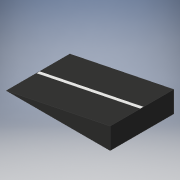
# Autodesk Inventor part: Ramp
Saved by Autodesk Inventor 2017 (Build 210142000, 142)
## iProperties
Created: 2017-04-14
Part Number: Ramp
Material: Generic
Document SubType Name: Modeling
Designer: Alex Tacescu
Density: 1 g/cm^3
Appearance: Rubber - Black
Author: Alex Tacescu
Autodesk Inventor part; units mm, degrees
ref_plane "YZ Plane" through (0, 0, 0) normal (1, 0, 0) x (0, 1, 0)
ref_plane "XZ Plane" through (0, 0, 0) normal (0, 1, 0) x (-1, 0, 0)
ref_plane "XY Plane" through (0, 0, 0) normal (0, 0, 1) x (1, 0, 0)
sketch "Sketch1" plane through (0, 0, 0) normal (0, 0, 1) x (1, 0, 0)
  line L0 (0, 0) -> (746.6045, 152.4)
  line L1 (0, 182.88) -> (0, -30.48) projected
  line L2 (-149.3209, 0) -> (895.9254, 0) projected
  line L3 (746.6045, 152.4) -> (746.6045, 0)
  line L4 (0, 0) -> (746.6045, 0)
  dimension "d0" = 152.4
  dimension "d1" = 762
  constraints: 6 end point, 1 perpendicular, 1 point on line, 1 vertical
  measures "d0" distance of L0.end L3.end
  measures "d1" distance of L0.start L0.end
extrude "Extrusion1" add sketch "Sketch1" along normal mid plane 457.2
sketch "Sketch4" plane through (0, 0, 228.6) normal (-0.2, 0.9798, 0) x (0.9798, 0.2, 0)
  line L0 (914.4, 228.6) -> (-152.4, 228.6) projected
  line L1 (762, 215.9) -> (0, 215.9)
  line L2 (0, 215.9) -> (0, 241.3)
  line L3 (0, 241.3) -> (762, 241.3)
  line L4 (762, 241.3) -> (762, 215.9)
  line L5 (762, 215.9) -> (0, 241.3) construction
  line L6 (0, 215.9) -> (762, 241.3) construction
  line L7 (0, 0) -> (0, 457.2) projected
  line L8 (762, 0) -> (0, 0) projected
  line L9 (762, 457.2) -> (762, 0) projected
  line L10 (0, 457.2) -> (762, 457.2) projected
  line L11 (762, 457.2) -> (762, 0) projected
  line L12 (0, 0) -> (0, 457.2) projected
  point P0 (0, 228.6)
  point P1 (381, 228.6)
  dimension "d6" = 25.4
  constraints: 12 end point, 3 midpoint, 2 collinear, 2 parallel, 1 horizontal, 1 perpendicular
  measures "d6" distance between parallel lines of L1 L3
extrude "Extrusion2" add sketch "Sketch4" along normal blind 0.254 contours L4 L1 L2 L0 | L0 L2 L3 L4
body "Solid1"
